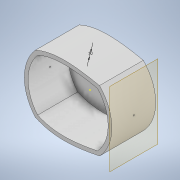
# Autodesk Inventor part: CameraHolder2
Saved by Autodesk Inventor 2021.1 (Build 251245010, 245A)
## iProperties
Created: 2023-07-02
Part Number: CameraHolder2
Material: Generic
Document SubType Name: Modeling
Designer: Drake
Density: 1 g/cm^3
Appearance: Default
Author: Drake
Autodesk Inventor part; units mm, degrees
ref_plane "XY Plane" through (0, 0, 0) normal (0, 0, 1) x (1, 0, 0)
sketch "Sketch1" plane through (0, 0, 0) normal (0, 0, 1) x (1, 0, 0)
  circle A0 centre (0, 0) radius 70
  line L0 (-52.3472, 46.4733) -> (-22.34, 60.3396) construction
  line L1 (-22.34, 60.3396) -> (10.9504, 56.7728) construction
  line L2 (10.9504, 56.7728) -> (50.2182, 48.7661) construction
  spline S0 degree 3 poles (-52.3472, 46.4733) (-22.34, 60.3396) (10.9504, 56.7728) (50.2182, 48.7661) knots 1 1 1 1 2 2 2 2
  line L3 (-70, 0) -> (70, 0)
  line L4 (-52.3472, -46.4733) -> (-22.34, -60.3396) construction
  line L5 (-22.34, -60.3396) -> (10.9504, -56.7728) construction
  line L6 (10.9504, -56.7728) -> (50.2182, -48.7661) construction
  spline S1 degree 3 poles (-52.3472, -46.4733) (-22.34, -60.3396) (10.9504, -56.7728) (50.2182, -48.7661) knots 1 1 1 1 2 2 2 2
  line L7 (0, 0) -> (0, 49.152)
  point P0 (50.2182, -48.7661)
  point P1 (0, 4.9536)
  point P2 (0, 5)
  point P3 (0.1096, -4.9988)
  point P4 (0.1096, 4.9988)
  dimension "d0" = 140
  dimension "d11" = 49.1519
  constraints: 4 end point, 4 point on circle, 4 symmetric about line, 1 centre point, 1 coincident, 1 horizontal, 1 vertical, 6 other
  measures "d0" diameter of A0
  measures "d11" distance of L7.start L7.end
sketch "Sketch2" plane through (0, 0, 0) normal (1, 0, 0) x (0, 1, 0)
  point P0 (0, 0)
extrude "Extrusion1" add sketch "Sketch1" against normal mid plane 70 contours L3 A0 S0 | A0 S1 L3
sketch "Sketch3" plane through (0, 0, 35) normal (0, 0, 1) x (1, 0, 0)
  spline S0 degree 3 poles (50.2182, 48.7661) (10.9504, 56.7728) (-22.34, 60.3396) (-52.3472, 46.4733) knots 0 0 0 0 1 1 1 1
  arc A0 (-52.3472, 46.4733) -> (-52.3472, -46.4733) centre (0, 0) ccw projected
  arc A1 (50.2182, -48.7661) -> (50.2182, 48.7661) centre (0, 0) ccw projected
  spline S1 degree 3 poles (-52.3472, -46.4733) (-22.34, -60.3396) (10.9504, -56.7728) (50.2182, -48.7661) knots 0 0 0 0 1 1 1 1
  arc A2 (47.1624, -43.2632) -> (47.1624, 43.2632) centre (0, 0) ccw
  arc A3 (-48.6797, 41.5486) -> (-48.6797, -41.5486) centre (0, 0) ccw
  spline S2 degree 5 poles (-48.6797, 41.5485) (-43.3248, 43.9315) (-37.7736, 45.8753) (-32.0737, 47.3484) (-19.8288, 49.5489) (-7.3905, 50.0535) (-0.8268, 49.9276) (12.7837, 49.0434) (26.2911, 47.1425) (33.2704, 45.9668) (40.2253, 44.6589) (47.1624, 43.2632) knots 0 0 0 0 0 0 0.300707 0.300707 0.300707 0.636966 0.636966 0.636966 1 1 1 1 1 1
  spline S3 degree 5 poles (47.1624, -43.2632) (40.2253, -44.6589) (33.2704, -45.9668) (26.2911, -47.1425) (12.7837, -49.0434) (-0.8268, -49.9276) (-7.3905, -50.0535) (-19.8288, -49.5489) (-32.0737, -47.3484) (-37.7736, -45.8753) (-43.3248, -43.9315) (-48.6797, -41.5485) knots 0 0 0 0 0 0 0.363034 0.363034 0.363034 0.699293 0.699293 0.699293 1 1 1 1 1 1
  dimension "d4" = 6
  constraints: 4 point on circle, 3 concentric, 2 centre point, 8 other
extrude "Extrusion2" cut sketch "Sketch3" against normal blind 64 contours S3 A3 S2 A2
ref_plane "Work Plane1" through (60, 0, 0) normal (1, 0, 0) x (0, 1, 0)
sketch "Sketch4" plane through (60, 0, 0) normal (1, 0, 0) x (0, 1, 0)
  circle A0 centre (0, 0) radius 1
  dimension "d8" = 2
  constraints: 1 centre point, 1 coincident
  measures "d8" diameter of A0
extrude "Extrusion3" cut sketch "Sketch4" against normal mid plane 300
ref_plane "Work Plane2" through (0, 49.152, 0) normal (0, 1, 0) x (-1, 0, 0)
sketch "Sketch5" plane through (0, 49.152, 0) normal (0, 1, 0) x (-1, 0, 0)
  circle A0 centre (0, 0) radius 5
  dimension "d13" = 10
  constraints: 1 centre point, 1 coincident
  measures "d13" diameter of A0
mirror "Mirror1" about plane through (0, 0, 0) normal (0, 0, 1) of "Extrusion3"
ref_plane "Work Plane3" through (70, 0, 0) normal (1, 0, 0) x (0, 1, 0)
equation "\"d2\" = d1"
equation "\"d1\" = 70"
body "Solid1"
